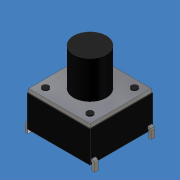
# Autodesk Inventor part: cRIO-FRC Switch
Saved by Autodesk Inventor 2011 (Build 150239000, 239)
## iProperties
Category: FRC Parts
Manager: Ed Sparks
Company: FirstCadLibrary
Shininess: 64.0
Length Units: 11272
Angle Units: 11279
Time Units: 11290
Mass Units: 11286
Length Display Precision: 3
Angle Display Precision: 2
Compacted: True
Part Number: cRIO-FRC Switch
Document SubType Name: Modeling
Created: 2005-12-26
Designer: Ed Sparks
Material: ABS Plastic
Project: FIRST
Engineer: Ed Sparks
Density: 1 g/cm^3
Density: 0.0
Volumn: 0.0
Area: 0.0
PropertySet Name: Model Information
Control State: 0
Master: False
Checked Out: False
Author: Ed Sparks
Keywords: FIRST
Autodesk Inventor part; units mm, degrees
ref_plane "YZ Plane" through (0, 0, 0) normal (1, 0, 0) x (0, 1, 0)
ref_plane "XZ Plane" through (0, 0, 0) normal (0, 1, 0) x (-1, 0, 0)
sketch "Sketch1" plane through (0, 0, 0) normal (0, 0, 1) x (1, 0, 0)
  line L0 (-3.175, 3.175) -> (3.175, 3.175)
  line L1 (3.175, 3.175) -> (3.175, -3.175)
  line L2 (3.175, -3.175) -> (-3.175, -3.175)
  line L3 (-3.175, -3.175) -> (-3.175, 3.175)
  line L4 (0, 0) -> (0, 0.9618)
  line L5 (0, 0) -> (0.9618, 0)
  dimension "d0" = 6.35
  constraints: 12 end point, 3 parallel, 3 perpendicular, 1 horizontal, 3 other
  measures "d0" distance of L0.start L0.end
extrude "Extrusion1" add sketch "Sketch1" along normal blind 3.175
sketch "Sketch2" plane through (0, 0, 3.175) normal (0, 0, 1) x (1, 0, 0)
  circle A0 centre (0, 0) radius 1.651
  dimension "d3" = 3.302
  constraints: 1 centre point
  measures "d3" diameter of A0
extrude "Extrusion2" add sketch "Sketch2" along normal blind 4.1656
sketch "Sketch3" plane through (0, 0, 3.175) normal (0, 0, 1) x (1, 0, 0)
  circle A0 centre (0, 0) radius 1.651 projected
  circle A1 centre (0, 0) radius 3.175
  line L0 (0, 0) -> (3.175, 3.175)
  circle A2 centre (2.2451, 2.2451) radius 0.3175
  dimension "d6" = 0.635
  constraints: 2 end point, 1 centre point, 1 coincident, 1 point on line, 3 other
  measures "d6" diameter of A2
extrude "Extrusion3" add sketch "Sketch3" along normal blind 0.508 contours A2 A1 L0 | L0 A1 A2 | L0 A2 A1 | A1 A2 L0
pattern_circular "Circular Pattern1" count 4 over 360 about axis through (0, 0, 3.175) along (0, 0, 1) of "Extrusion3"
sketch "Sketch4" plane through (0, 0, 3.175) normal (0, 0, 1) x (1, 0, 0)
  circle A0 centre (2.2451, -2.2451) radius 0.3175 projected
  circle A1 centre (-2.2451, -2.2451) radius 0.3175 projected
  circle A2 centre (-2.2451, 2.2451) radius 0.3175 projected
  circle A3 centre (2.2451, 2.2451) radius 0.3175 projected
  circle A4 centre (0, 0) radius 1.651 projected
  line L0 (3.175, 3.175) -> (3.175, -3.175) projected
  line L1 (-3.175, 3.175) -> (3.175, 3.175) projected
  line L2 (-3.175, -3.175) -> (-3.175, 3.175) projected
  line L3 (3.175, -3.175) -> (-3.175, -3.175) projected
  line L4 (3.1021, 3.1021) -> (3.1021, -3.1021)
  line L5 (3.1021, -3.1021) -> (-3.1021, -3.1021)
  line L6 (-3.1021, -3.1021) -> (-3.1021, 3.1021)
  line L7 (-3.1021, 3.1021) -> (3.1021, 3.1021)
  constraints: 8 end point, 3 other
extrude "Extrusion4" add sketch "Sketch4" along normal blind 0.381 contours L4 L5 L6 L7
sketch "Sketch5" plane through (-3.175, -3.175, 0) normal (0, -1, 0) x (1, 0, 0)
  line L0 (0, 0) -> (0, 3.175) projected
  line L1 (6.35, 0) -> (0, 0) projected
  line L2 (0.127, 0.508) -> (0.508, 0.508)
  line L3 (0.508, 0.508) -> (0.508, 0.254)
  line L4 (0.508, 0.254) -> (0.127, 0.254)
  line L5 (0.127, 0.254) -> (0.127, 0.508)
  dimension "d14" = 0.381
  dimension "d15" = 0.254
  dimension "d16" = 0.127
  dimension "d17" = 0.254
  constraints: 8 end point, 2 parallel, 1 horizontal, 1 perpendicular
  measures "d14" distance of L2.start L2.end
  measures "d15" distance of L2.end L3.end
  measures "d16" distance between parallel lines of L0 L5
  measures "d17" distance between parallel lines of L1 L4
ref_plane "Work Plane1" through (-2.667, -3.175, 0.508) normal (-1, 0, 0) x (0, 0, -1)
sketch "Sketch6" plane through (-2.667, -3.175, 0.508) normal (-1, 0, 0) x (0, 0, -1)
  line L0 (0, -0.1801) -> (0, 0.0739)
  line L1 (0.254, 0.3279) -> (1.016, 0.3279)
  arc A0 (0.254, 0.3279) -> (0, 0.0739) centre (0.254, 0.0739) ccw
  point P0 (0, 0.3279)
  dimension "d19" = 0.508
  dimension "d20" = 1.016
  dimension "d21" = 0.254
  constraints: 4 end point, 2 point on circle, 2 point on line, 2 tangent, 1 centre point, 1 perpendicular, 1 vertical
  measures "d19" distance of L0.start point (0, 0.328)
  measures "d20" distance of point (0, 0.328) L1.end
  measures "d21" radius of A0
sweep "Sweep1" add profiles "Sketch5" path "Sketch6"
mirror "Mirror1" about plane through (0, 0, 0) normal (1, 0, 0) of "Sweep1"
mirror "Mirror2" about plane through (0, 0, 0) normal (0, 1, 0) of "Sweep1", "Mirror1"
body "Solid1"
